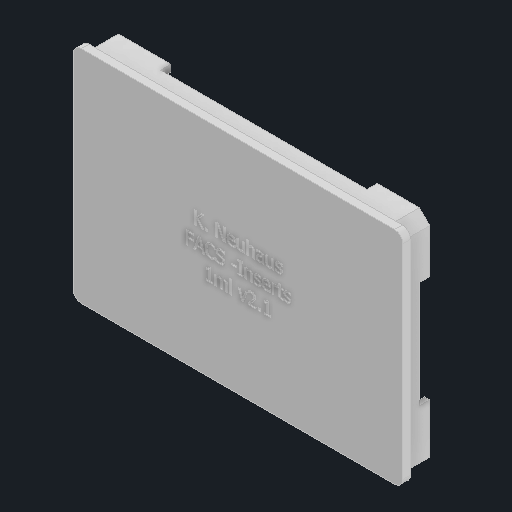
# Autodesk Inventor part: Holder_FACS_1mL_Petridish
Saved by Autodesk Inventor 2026 (Build 300175050, 175E)
## iProperties
Created: 2024-09-30
Part Number: Holder_FACS_1mL_Petridish
Material: Generisch
Document SubType Name: Modeling
Designer: neuhau0004
Density: 1 g/cm^3
Appearance: Vorgabe
Author: neuhau0004
Autodesk Inventor part; units mm, degrees
ref_plane "YZ Plane" through (0, 0, 0) normal (1, 0, 0) x (0, 1, 0)
ref_plane "XZ Plane" through (0, 0, 0) normal (0, 1, 0) x (-1, 0, 0)
ref_plane "XY Plane" through (0, 0, 0) normal (0, 0, 1) x (1, 0, 0)
sketch "Skizze1" plane through (0, 0, 0) normal (0, 0, 1) x (1, 0, 0)
  line L0 (-62.3, -42.74) -> (62.3, -42.74)
  line L1 (62.3, -42.74) -> (62.3, 42.74)
  line L2 (62.3, 42.74) -> (-62.3, 42.74)
  line L3 (-62.3, 42.74) -> (-62.3, -42.74)
  line L4 (-62.3, -42.74) -> (62.3, 42.74) construction
  line L5 (62.3, -42.74) -> (-62.3, 42.74) construction
  line L6 (-60.7, 42.74) -> (60.7, 42.74)
  line L7 (63.88, 39.56) -> (63.88, -39.56)
  line L8 (60.7, -42.74) -> (-60.7, -42.74)
  line L9 (-63.88, -39.56) -> (-63.88, 39.56)
  line L10 (-63.88, 42.74) -> (63.88, -42.74) construction
  line L11 (63.88, 42.74) -> (-63.88, -42.74) construction
  circle A0 centre (-40, 19.74) radius 18.45
  circle A1 centre (0, 19.74) radius 18.45
  circle A2 centre (40, 19.74) radius 18.45
  circle A3 centre (-40, -19.26) radius 18.45
  circle A4 centre (0, -19.26) radius 18.45
  circle A5 centre (40, -19.26) radius 18.45
  arc A6 (63.88, 39.56) -> (60.7, 42.74) centre (60.7, 39.56) ccw
  arc A7 (60.7, -42.74) -> (63.88, -39.56) centre (60.7, -39.56) ccw
  arc A8 (-63.88, -39.56) -> (-60.7, -42.74) centre (-60.7, -39.56) ccw
  arc A9 (-60.7, 42.74) -> (-63.88, 39.56) centre (-60.7, 39.56) ccw
  line L12 (-60.3, 40.85) -> (60.3, 40.85)
  line L13 (60.3, 40.85) -> (60.3, -40.85)
  line L14 (60.3, -40.85) -> (-60.3, -40.85)
  line L15 (-60.3, -40.85) -> (-60.3, 40.85)
  line L16 (-60.3, 40.85) -> (60.3, -40.85) construction
  line L17 (60.3, 40.85) -> (-60.3, -40.85) construction
  ellipse E0 centre (40, 19.74) end of major axis (24, 37.44) minor radius 11.9962
  ellipse E1 centre (0, 19.74) end of major axis (-16, 37.44) minor radius 11.9962
  ellipse E2 centre (-40, 19.74) end of major axis (-56, 37.44) minor radius 11.9962
  ellipse E3 centre (40, -19.26) end of major axis (24, -1.56) minor radius 11.9962
  ellipse E4 centre (0, -19.26) end of major axis (-16, -1.56) minor radius 11.9962
  ellipse E5 centre (-40, -19.26) end of major axis (-56, -1.56) minor radius 11.9962
  line L18 (-40, 40.85) -> (-60.3, 40.85)
  line L19 (-60.3, 40.85) -> (-60.3, 19.74)
  line L20 (-58.45, 19.74) -> (-60.3, 19.74)
  line L21 (-58.45, -19.26) -> (-60.3, -19.26)
  line L22 (-60.3, -40.85) -> (-60.3, -19.26)
  line L23 (-40, -37.71) -> (-40, -40.85)
  line L24 (-60.3, -40.85) -> (-40, -40.85)
  arc A10 (-40, 38.19) -> (-58.45, 19.74) centre (-40, 19.74) ccw
  line L25 (-40, 40.85) -> (-40, 38.19)
  line L26 (40, 38.19) -> (40, 40.85)
  line L27 (58.45, 19.74) -> (60.3, 19.74)
  line L28 (58.45, -19.26) -> (60.3, -19.26)
  line L29 (40, -37.71) -> (40, -40.85)
  line L30 (-60.3, -19.26) -> (-60.3, -21.66)
  line L31 (-60.3, -21.66) -> (-58.2932, -21.66)
  line L32 (60.3, -21.66) -> (58.2932, -21.66)
  point P0 (0, 0)
  point P1 (-60.7, 42.74)
  point P2 (60.7, -42.74)
  point P3 (-22.5977, -25.3889)
  point P4 (-35.6534, -37.1907)
  point P5 (-57.4023, -13.1311)
  point P6 (-44.3466, -1.3293)
  point P7 (17.4023, -25.3889)
  point P8 (4.3466, -37.1907)
  point P9 (-17.4023, -13.1311)
  point P10 (-4.3466, -1.3293)
  point P11 (57.4023, -25.3889)
  point P12 (44.3466, -37.1907)
  point P13 (22.5977, -13.1311)
  point P14 (35.6534, -1.3293)
  point P15 (-22.5977, 13.6111)
  point P16 (-35.6534, 1.8093)
  point P17 (-57.4023, 25.8689)
  point P18 (-44.3466, 37.6707)
  point P19 (17.4023, 13.6111)
  point P20 (4.3466, 1.8093)
  point P21 (-17.4023, 25.8689)
  point P22 (-4.3466, 37.6707)
  point P23 (57.4023, 13.6111)
  point P24 (44.3466, 1.8093)
  point P25 (22.5977, 25.8689)
  point P26 (35.6534, 37.6707)
  point P27 (62.3, 42.3082)
  point P28 (62.3, -42.3082)
  point P29 (-62.3, -42.3082)
  point P30 (-62.3, 42.3082)
  dimension "d0" = 124.6
  dimension "d1" = 85.48
  dimension "d2" = 127.76
  dimension "d3" = 85.48
  dimension "d9" = 36.9
  dimension "d10" = 22.3
  dimension "d13" = 40
  dimension "d16" = 39
  dimension "d19" = 23
  dimension "d20" = 3.18
  dimension "d21" = 3.18
  dimension "d24" = 120.6
  dimension "d25" = 81.7
  dimension "d28" = 40
  dimension "d31" = 39
  dimension "d54" = 2.4
  dimension "d55" = 3.18
  constraints: 66 end point, 20 point on circle, 18 point on line, 13 perpendicular, 11 centre point, 8 tangent, 7 horizontal, 6 midpoint, 6 parallel, 6 vertical, 2 coincident, 2 collinear, 2 equal radius, 27 other
  measures "d0" distance of L2.end L1.end
  measures "d1" distance of L1.end L0.end
  measures "d2" distance of L10.end L11.end
  measures "d3" distance of L11.start L10.end
  measures "d9" diameter of A0
  measures "d10" distance from line of L3 A0.centre
  measures "d13" distance of A0.centre A1.centre
  measures "d16" distance of A0.centre A3.centre
  measures "d19" distance from line of L2 A0.centre
  measures "d20" radius of A6
  measures "d21" radius of A8
  measures "d24" distance of L13.end L14.end
  measures "d25" distance of L12.end L13.end
  measures "d28" distance of point (40, 19.74) point (0, 19.74)
  measures "d31" distance of point (40, 19.74) point (40, -19.26)
  measures "d54" distance of L21.end L30.end
  measures "d55" radius of A9
extrude "Extrusion1" add sketch "Skizze1" along normal blind 3 contours A8 L3 A9 L2 A6 L1 A7 L0 | A8 L9 A9 L3 | L1 A6 L7 A7 | A0 E2 | A0 L25 L12 L26 A2 E0 L27 L13 L28 A5 E3 L29 L14 L23 A3 E5 L21 L15 L20 E2 | A0 E2 L20 L15 L12 L25 | E2 A0 | A0 E2 | A0 E2 | A0 E2 | L12 L13 L27 A2 L26 | A2 E0 | L21 A3 L31 L15 | E0 A2 | A2 E0 | L31 A3 L23 L14 L15 | A3 E5 | L13 L32 A5 L28 | E0 A2 | E0 A2 | E5 A3 | A3 E5 | L13 L14 L29 A5 E3 L32 | A5 E3 | A3 E5 | A3 E5 | E3 A5 | A5 E3 | E3 A5 | E3 A5 | A1 E1 | E1 A1 | A1 E1 | E1 A1 | E1 A1 | A4 E4 | E4 A4 | A4 E4 | E4 A4 | E4 A4
extrude "Extrusion2" add sketch "Skizze1" against normal blind 7 contours A0 L25 L12 L26 A2 E0 L27 L13 L28 A5 E3 L29 L14 L23 A3 E5 L21 L15 L20 E2 | A0 E2 L20 L15 L12 L25 | L12 L13 L27 A2 L26 | L21 A3 L31 L15 | L31 A3 L23 L14 L15 | L13 L32 A5 L28 | L13 L14 L29 A5 E3 L32
fillet "Rundung1" radius 2 3 edges at (60.3, -40.85, -3.5) (-60.3, -40.85, -3.5) (-60.3, 40.85, -3.5)
chamfer "Fase1" distance 1 angle 45 24 edges at (-24, 2.04, -7) (-56, 37.44, -7) (-53.6868, 7.3677, -7) (-26.3132, 32.1123, -7) (-56, -1.56, -7) (-24, -36.96, -7) (-26.3132, -6.8877, -7) (-53.6868, -31.6323, -7) (-16, 37.44, -7) (16, 2.04, -7) (-13.6868, 7.3677, -7) (13.6868, 32.1123, -7) (-16, -1.56, -7) (16, -36.96, -7) (-13.6868, -31.6323, -7) (13.6868, -6.8877, -7) (24, 37.44, -7) (56, 2.04, -7) (26.3132, 7.3677, -7) (53.6868, 32.1123, -7) (24, -1.56, -7) (56, -36.96, -7) (53.6868, -6.8877, -7) (26.3132, -31.6323, -7)
chamfer "Fase2" distance 4 angle 45 1 edges at (60.3, 40.85, -3.5)
sketch "Skizze3" plane through (0, 0, 3) normal (0, 0, 1) x (1, 0, 0)
  line L0 (-25.4173, 12.5) -> (25.4173, 12.5) construction
  line L1 (25.4173, 12.5) -> (25.4173, -12.5) construction
  line L2 (25.4173, -12.5) -> (-25.4173, -12.5) construction
  line L3 (-25.4173, -12.5) -> (-25.4173, 12.5) construction
  line L4 (-13.1767, 5.6209) -> (-14.0397, 5.6209)
  line L5 (-14.0397, 5.6209) -> (-15.8671, 7.9467)
  line L6 (-15.8671, 7.9467) -> (-16.1588, 7.6185)
  line L7 (-16.1588, 7.6185) -> (-16.1588, 5.6209)
  line L8 (-16.1588, 5.6209) -> (-16.8233, 5.6209)
  line L9 (-16.8233, 5.6209) -> (-16.8233, 10.6209)
  line L10 (-16.8233, 10.6209) -> (-16.1588, 10.6209)
  line L11 (-16.1588, 10.6209) -> (-16.1588, 8.3235)
  line L12 (-16.1588, 8.3235) -> (-14.1086, 10.6209)
  line L13 (-14.1086, 10.6209) -> (-13.2982, 10.6209)
  line L14 (-13.2982, 10.6209) -> (-15.3687, 8.3884)
  line L15 (-15.3687, 8.3884) -> (-13.1767, 5.6209)
  line L16 (-11.8476, 5.6209) -> (-12.6499, 5.6209)
  line L17 (-12.6499, 5.6209) -> (-12.6499, 6.5772)
  line L18 (-12.6499, 6.5772) -> (-11.8476, 6.5772)
  line L19 (-11.8476, 6.5772) -> (-11.8476, 5.6209)
  line L20 (-4.9716, 5.6209) -> (-5.7172, 5.6209)
  line L21 (-5.7172, 5.6209) -> (-7.9295, 9.9321)
  line L22 (-7.9295, 9.9321) -> (-7.9295, 5.6209)
  line L23 (-7.9295, 5.6209) -> (-8.5494, 5.6209)
  line L24 (-8.5494, 5.6209) -> (-8.5494, 10.6209)
  line L25 (-8.5494, 10.6209) -> (-7.6053, 10.6209)
  line L26 (-7.6053, 10.6209) -> (-5.5916, 6.6623)
  line L27 (-5.5916, 6.6623) -> (-5.5916, 10.6209)
  line L28 (-5.5916, 10.6209) -> (-4.9716, 10.6209)
  line L29 (-4.9716, 10.6209) -> (-4.9716, 5.6209)
  spline S0 degree 2 poles (-2.3784, 5.5359) (-3.278, 5.5359) (-4.2666, 6.5448) (-4.2666, 7.4767) knots 0 0 0 1 2 2 2
  spline S1 degree 2 poles (-4.2666, 7.4767) (-4.2666, 8.3924) (-3.3063, 9.4783) (-2.5324, 9.4783) knots 0 0 0 1 2 2 2
  spline S2 degree 2 poles (-2.5324, 9.4783) (-2.184, 9.4783) (-1.6451, 9.2757) (-1.4465, 9.061) knots 0 0 0 1 2 2 2
  spline S3 degree 2 poles (-1.4465, 9.061) (-1.2439, 8.8462) (-1.0292, 8.2263) (-1.0292, 7.7765) knots 0 0 0 1 2 2 2
  line L30 (-1.0292, 7.7765) -> (-1.0292, 7.4321)
  line L31 (-1.0292, 7.4321) -> (-3.6264, 7.4321)
  spline S4 degree 2 poles (-3.6264, 7.4321) (-3.6264, 6.7798) (-2.97, 6.0869) (-2.3865, 6.0869) knots 0 0 0 1 2 2 2
  spline S5 degree 2 poles (-2.3865, 6.0869) (-2.1799, 6.0869) (-1.7788, 6.1801) (-1.6167, 6.253) knots 0 0 0 1 2 2 2
  spline S6 degree 2 poles (-1.6167, 6.253) (-1.4465, 6.3341) (-1.2115, 6.4759) (-1.1345, 6.5407) knots 0 0 0 1 2 2 2
  line L32 (-1.1345, 6.5407) -> (-1.0981, 6.5407)
  line L33 (-1.0981, 6.5407) -> (-1.0981, 5.8519)
  spline S7 degree 2 poles (-1.0981, 5.8519) (-1.2075, 5.8073) (-1.5397, 5.6777) (-1.6694, 5.6412) knots 0 0 0 1 2 2 2
  spline S8 degree 2 poles (-1.6694, 5.6412) (-1.8517, 5.5885) (-2.1515, 5.5359) (-2.3784, 5.5359) knots 0 0 0 1 2 2 2
  spline S9 degree 2 poles (-1.6451, 7.9143) (-1.6532, 8.1696) (-1.7585, 8.5423) (-1.8598, 8.6679) knots 0 0 0 1 2 2 2
  spline S10 degree 2 poles (-1.8598, 8.6679) (-1.9692, 8.8098) (-2.3136, 8.9597) (-2.5689, 8.9597) knots 0 0 0 1 2 2 2
  spline S11 degree 2 poles (-2.5689, 8.9597) (-2.8201, 8.9597) (-3.1726, 8.8098) (-3.3185, 8.6639) knots 0 0 0 1 2 2 2
  spline S12 degree 2 poles (-3.3185, 8.6639) (-3.4603, 8.514) (-3.6062, 8.1534) (-3.6264, 7.9143) knots 0 0 0 1 2 2 2
  line L34 (-3.6264, 7.9143) -> (-1.6451, 7.9143)
  line L35 (2.5284, 5.6209) -> (1.8963, 5.6209)
  line L36 (1.8963, 5.6209) -> (1.8963, 6.0342)
  spline S13 degree 2 poles (1.8963, 6.0342) (1.6045, 5.779) (1.0818, 5.5156) (0.7577, 5.5156) knots 0 0 0 1 2 2 2
  spline S14 degree 2 poles (0.7577, 5.5156) (0.5146, 5.5156) (0.081, 5.6777) (-0.077, 5.8519) knots 0 0 0 1 2 2 2
  spline S15 degree 2 poles (-0.077, 5.8519) (-0.2391, 6.0261) (-0.4173, 6.5569) (-0.4173, 6.9378) knots 0 0 0 1 2 2 2
  line L37 (-0.4173, 6.9378) -> (-0.4173, 9.373)
  line L38 (-0.4173, 9.373) -> (0.2147, 9.373)
  line L39 (0.2147, 9.373) -> (0.2147, 7.2336)
  spline S16 degree 2 poles (0.2147, 7.2336) (0.2147, 6.9337) (0.2593, 6.5407) (0.3363, 6.3948) knots 0 0 0 1 2 2 2
  spline S17 degree 2 poles (0.3363, 6.3948) (0.4133, 6.249) (0.6767, 6.1153) (0.9238, 6.1153) knots 0 0 0 1 2 2 2
  spline S18 degree 2 poles (0.9238, 6.1153) (1.1548, 6.1153) (1.6775, 6.3786) (1.8963, 6.5691) knots 0 0 0 1 2 2 2
  line L40 (1.8963, 6.5691) -> (1.8963, 9.373)
  line L41 (1.8963, 9.373) -> (2.5284, 9.373)
  line L42 (2.5284, 9.373) -> (2.5284, 5.6209)
  line L43 (6.3898, 5.6209) -> (5.7577, 5.6209)
  line L44 (5.7577, 5.6209) -> (5.7577, 7.7603)
  spline S19 degree 2 poles (5.7577, 7.7603) (5.7577, 8.0196) (5.7091, 8.4654) (5.6361, 8.5991) knots 0 0 0 1 2 2 2
  spline S20 degree 2 poles (5.6361, 8.5991) (5.5592, 8.7409) (5.2836, 8.8786) (5.0486, 8.8786) knots 0 0 0 1 2 2 2
  spline S21 degree 2 poles (5.0486, 8.8786) (4.8136, 8.8786) (4.3152, 8.6274) (4.0762, 8.4248) knots 0 0 0 1 2 2 2
  line L45 (4.0762, 8.4248) -> (4.0762, 5.6209)
  line L46 (4.0762, 5.6209) -> (3.4441, 5.6209)
  line L47 (3.4441, 5.6209) -> (3.4441, 10.8438)
  line L48 (3.4441, 10.8438) -> (4.0762, 10.8438)
  line L49 (4.0762, 10.8438) -> (4.0762, 8.9556)
  spline S22 degree 2 poles (4.0762, 8.9556) (4.3598, 9.2109) (4.9068, 9.4783) (5.2147, 9.4783) knots 0 0 0 1 2 2 2
  spline S23 degree 2 poles (5.2147, 9.4783) (5.7658, 9.4783) (6.3898, 8.749) (6.3898, 8.0561) knots 0 0 0 1 2 2 2
  line L50 (6.3898, 8.0561) -> (6.3898, 5.6209)
  spline S24 degree 2 poles (9.3679, 6.018) (9.2909, 5.9613) (9.0316, 5.7587) (8.91, 5.6979) knots 0 0 0 1 2 2 2
  spline S25 degree 2 poles (8.91, 5.6979) (8.7439, 5.6088) (8.4319, 5.5156) (8.1483, 5.5156) knots 0 0 0 1 2 2 2
  spline S26 degree 2 poles (8.1483, 5.5156) (7.9173, 5.5156) (7.5, 5.6898) (7.342, 5.8478) knots 0 0 0 1 2 2 2
  spline S27 degree 2 poles (7.342, 5.8478) (7.1921, 6.0018) (7.0097, 6.4556) (7.0097, 6.7068) knots 0 0 0 1 2 2 2
  spline S28 degree 2 poles (7.0097, 6.7068) (7.0097, 7.0958) (7.3379, 7.6469) (7.6945, 7.8049) knots 0 0 0 1 2 2 2
  spline S29 degree 2 poles (7.6945, 7.8049) (8.0105, 7.9508) (8.8695, 8.0602) (9.3679, 8.0885) knots 0 0 0 1 2 2 2
  line L51 (9.3679, 8.0885) -> (9.3679, 8.2101)
  spline S30 degree 2 poles (9.3679, 8.2101) (9.3679, 8.4289) (9.2342, 8.7004) (9.1126, 8.7773) knots 0 0 0 1 2 2 2
  spline S31 degree 2 poles (9.1126, 8.7773) (8.9911, 8.8543) (8.6426, 8.903) (8.4562, 8.903) knots 0 0 0 1 2 2 2
  spline S32 degree 2 poles (8.4562, 8.903) (8.2374, 8.903) (7.6459, 8.7733) (7.3501, 8.6477) knots 0 0 0 1 2 2 2
  line L52 (7.3501, 8.6477) -> (7.3136, 8.6477)
  line L53 (7.3136, 8.6477) -> (7.3136, 9.2919)
  spline S33 degree 2 poles (7.3136, 9.2919) (7.4878, 9.3406) (8.1402, 9.4621) (8.4603, 9.4621) knots 0 0 0 1 2 2 2
  spline S34 degree 2 poles (8.4603, 9.4621) (8.8493, 9.4621) (9.3801, 9.3406) (9.5908, 9.1825) knots 0 0 0 1 2 2 2
  spline S35 degree 2 poles (9.5908, 9.1825) (9.7974, 9.0286) (10, 8.5383) (10, 8.1858) knots 0 0 0 1 2 2 2
  line L54 (10, 8.1858) -> (10, 5.6209)
  line L55 (10, 5.6209) -> (9.3679, 5.6209)
  line L56 (9.3679, 5.6209) -> (9.3679, 6.018)
  line L57 (9.3679, 6.5448) -> (9.3679, 7.5861)
  spline S36 degree 2 poles (9.3679, 7.5861) (9.141, 7.5658) (8.4562, 7.497) (8.2415, 7.4321) knots 0 0 0 1 2 2 2
  spline S37 degree 2 poles (8.2415, 7.4321) (7.9903, 7.3551) (7.6621, 7.035) (7.6621, 6.7514) knots 0 0 0 1 2 2 2
  spline S38 degree 2 poles (7.6621, 6.7514) (7.6621, 6.4273) (8.0267, 6.0991) (8.3752, 6.0991) knots 0 0 0 1 2 2 2
  spline S39 degree 2 poles (8.3752, 6.0991) (8.671, 6.0991) (9.1572, 6.3543) (9.3679, 6.5448) knots 0 0 0 1 2 2 2
  line L58 (13.8047, 5.6209) -> (13.1726, 5.6209)
  line L59 (13.1726, 5.6209) -> (13.1726, 6.0342)
  spline S40 degree 2 poles (13.1726, 6.0342) (12.8809, 5.779) (12.3582, 5.5156) (12.034, 5.5156) knots 0 0 0 1 2 2 2
  spline S41 degree 2 poles (12.034, 5.5156) (11.7909, 5.5156) (11.3574, 5.6777) (11.1994, 5.8519) knots 0 0 0 1 2 2 2
  spline S42 degree 2 poles (11.1994, 5.8519) (11.0373, 6.0261) (10.859, 6.5569) (10.859, 6.9378) knots 0 0 0 1 2 2 2
  line L60 (10.859, 6.9378) -> (10.859, 9.373)
  line L61 (10.859, 9.373) -> (11.4911, 9.373)
  line L62 (11.4911, 9.373) -> (11.4911, 7.2336)
  spline S43 degree 2 poles (11.4911, 7.2336) (11.4911, 6.9337) (11.5357, 6.5407) (11.6126, 6.3948) knots 0 0 0 1 2 2 2
  spline S44 degree 2 poles (11.6126, 6.3948) (11.6896, 6.249) (11.953, 6.1153) (12.2002, 6.1153) knots 0 0 0 1 2 2 2
  spline S45 degree 2 poles (12.2002, 6.1153) (12.4311, 6.1153) (12.9538, 6.3786) (13.1726, 6.5691) knots 0 0 0 1 2 2 2
  line L63 (13.1726, 6.5691) -> (13.1726, 9.373)
  line L64 (13.1726, 9.373) -> (13.8047, 9.373)
  line L65 (13.8047, 9.373) -> (13.8047, 5.6209)
  spline S46 degree 2 poles (15.7334, 5.5318) (15.3566, 5.5318) (14.7042, 5.7344) (14.4895, 5.8478) knots 0 0 0 1 2 2 2
  line L66 (14.4895, 5.8478) -> (14.4895, 6.5569)
  line L67 (14.4895, 6.5569) -> (14.5219, 6.5569)
  spline S47 degree 2 poles (14.5219, 6.5569) (14.6029, 6.4921) (14.8217, 6.3381) (15.0041, 6.253) knots 0 0 0 1 2 2 2
  spline S48 degree 2 poles (15.0041, 6.253) (15.1621, 6.176) (15.5511, 6.0626) (15.7577, 6.0626) knots 0 0 0 1 2 2 2
  spline S49 degree 2 poles (15.7577, 6.0626) (15.9076, 6.0626) (16.252, 6.1315) (16.3331, 6.1882) knots 0 0 0 1 2 2 2
  spline S50 degree 2 poles (16.3331, 6.1882) (16.4506, 6.2652) (16.5559, 6.4394) (16.5559, 6.6177) knots 0 0 0 1 2 2 2
  spline S51 degree 2 poles (16.5559, 6.6177) (16.5559, 6.8406) (16.3128, 7.0715) (16.0008, 7.1485) knots 0 0 0 1 2 2 2
  spline S52 degree 2 poles (16.0008, 7.1485) (15.8793, 7.1769) (15.4903, 7.2579) (15.3241, 7.3025) knots 0 0 0 1 2 2 2
  spline S53 degree 2 poles (15.3241, 7.3025) (14.8947, 7.4281) (14.5057, 7.9467) (14.5057, 8.3154) knots 0 0 0 1 2 2 2
  spline S54 degree 2 poles (14.5057, 8.3154) (14.5057, 8.826) (15.2715, 9.4621) (15.9036, 9.4621) knots 0 0 0 1 2 2 2
  spline S55 degree 2 poles (15.9036, 9.4621) (16.2156, 9.4621) (16.8477, 9.3081) (17.0624, 9.1906) knots 0 0 0 1 2 2 2
  line L68 (17.0624, 9.1906) -> (17.0624, 8.514)
  line L69 (17.0624, 8.514) -> (17.03, 8.514)
  spline S56 degree 2 poles (17.03, 8.514) (16.7869, 8.7085) (16.1953, 8.9313) (15.8914, 8.9313) knots 0 0 0 1 2 2 2
  spline S57 degree 2 poles (15.8914, 8.9313) (15.5794, 8.9313) (15.1499, 8.6679) (15.1499, 8.4046) knots 0 0 0 1 2 2 2
  spline S58 degree 2 poles (15.1499, 8.4046) (15.1499, 8.1655) (15.4052, 7.9346) (15.6888, 7.8616) knots 0 0 0 1 2 2 2
  spline S59 degree 2 poles (15.6888, 7.8616) (15.8266, 7.8252) (16.175, 7.7522) (16.3655, 7.7077) knots 0 0 0 1 2 2 2
  spline S60 degree 2 poles (16.3655, 7.7077) (16.7788, 7.6023) (17.2002, 7.1201) (17.2002, 6.7028) knots 0 0 0 1 2 2 2
  spline S61 degree 2 poles (17.2002, 6.7028) (17.2002, 6.4597) (17.0097, 6.0302) (16.8233, 5.8722) knots 0 0 0 1 2 2 2
  spline S62 degree 2 poles (16.8233, 5.8722) (16.6248, 5.706) (16.1183, 5.5318) (15.7334, 5.5318) knots 0 0 0 1 2 2 2
  line L70 (-17.1252, 1.797) -> (-19.451, 1.797)
  line L71 (-19.451, 1.797) -> (-19.451, 0.387)
  line L72 (-19.451, 0.387) -> (-17.2224, 0.387)
  line L73 (-17.2224, 0.387) -> (-17.2224, -0.2046)
  line L74 (-17.2224, -0.2046) -> (-19.451, -0.2046)
  line L75 (-19.451, -0.2046) -> (-19.451, -2.6114)
  line L76 (-19.451, -2.6114) -> (-20.1155, -2.6114)
  line L77 (-20.1155, -2.6114) -> (-20.1155, 2.3886)
  line L78 (-20.1155, 2.3886) -> (-17.1252, 2.3886)
  line L79 (-17.1252, 2.3886) -> (-17.1252, 1.797)
  line L80 (-17.0685, -2.6114) -> (-15.3829, 2.3886)
  line L81 (-15.3829, 2.3886) -> (-14.5644, 2.3886)
  line L82 (-14.5644, 2.3886) -> (-12.8788, -2.6114)
  line L83 (-12.8788, -2.6114) -> (-13.5798, -2.6114)
  line L84 (-13.5798, -2.6114) -> (-14.0336, -1.2135)
  line L85 (-14.0336, -1.2135) -> (-15.9421, -1.2135)
  line L86 (-15.9421, -1.2135) -> (-16.3959, -2.6114)
  line L87 (-16.3959, -2.6114) -> (-17.0685, -2.6114)
  line L88 (-14.216, -0.6463) -> (-14.9899, 1.7079)
  line L89 (-14.9899, 1.7079) -> (-15.7597, -0.6463)
  line L90 (-15.7597, -0.6463) -> (-14.216, -0.6463)
  spline S63 degree 2 poles (-10.4518, -2.7006) (-10.938, -2.7006) (-11.7605, -2.3724) (-12.0604, -2.0442) knots 0 0 0 1 2 2 2
  spline S64 degree 2 poles (-12.0604, -2.0442) (-12.3602, -1.72) (-12.6884, -0.7476) (-12.6884, -0.1155) knots 0 0 0 1 2 2 2
  spline S65 degree 2 poles (-12.6884, -0.1155) (-12.6884, 0.5126) (-12.3683, 1.4445) (-12.0644, 1.7889) knots 0 0 0 1 2 2 2
  spline S66 degree 2 poles (-12.0644, 1.7889) (-11.7646, 2.1252) (-10.9461, 2.4777) (-10.4396, 2.4777) knots 0 0 0 1 2 2 2
  spline S67 degree 2 poles (-10.4396, 2.4777) (-10.1884, 2.4777) (-9.7468, 2.4048) (-9.5604, 2.3481) knots 0 0 0 1 2 2 2
  spline S68 degree 2 poles (-9.5604, 2.3481) (-9.3983, 2.2954) (-9.062, 2.1455) (-8.8959, 2.0563) knots 0 0 0 1 2 2 2
  line L91 (-8.8959, 2.0563) -> (-8.8959, 1.2541)
  line L92 (-8.8959, 1.2541) -> (-8.9485, 1.2541)
  spline S69 degree 2 poles (-8.9485, 1.2541) (-9.0377, 1.3351) (-9.3132, 1.562) (-9.5117, 1.6714) knots 0 0 0 1 2 2 2
  spline S70 degree 2 poles (-9.5117, 1.6714) (-9.7022, 1.7767) (-10.1519, 1.9105) (-10.4437, 1.9105) knots 0 0 0 1 2 2 2
  spline S71 degree 2 poles (-10.4437, 1.9105) (-10.7638, 1.9105) (-11.3351, 1.6471) (-11.5498, 1.3959) knots 0 0 0 1 2 2 2
  spline S72 degree 2 poles (-11.5498, 1.3959) (-11.7605, 1.1406) (-11.9955, 0.3667) (-11.9955, -0.1155) knots 0 0 0 1 2 2 2
  spline S73 degree 2 poles (-11.9955, -0.1155) (-11.9955, -0.6301) (-11.7484, -1.3716) (-11.5336, -1.6268) knots 0 0 0 1 2 2 2
  spline S74 degree 2 poles (-11.5336, -1.6268) (-11.3229, -1.874) (-10.7597, -2.1252) (-10.4437, -2.1252) knots 0 0 0 1 2 2 2
  spline S75 degree 2 poles (-10.4437, -2.1252) (-10.156, -2.1252) (-9.6657, -1.9834) (-9.4753, -1.878) knots 0 0 0 1 2 2 2
  spline S76 degree 2 poles (-9.4753, -1.878) (-9.2929, -1.7727) (-9.0215, -1.5539) (-8.9445, -1.4769) knots 0 0 0 1 2 2 2
  line L93 (-8.9445, -1.4769) -> (-8.8959, -1.4769)
  line L94 (-8.8959, -1.4769) -> (-8.8959, -2.2711)
  spline S77 degree 2 poles (-8.8959, -2.2711) (-9.062, -2.3481) (-9.3537, -2.4899) (-9.5604, -2.5547) knots 0 0 0 1 2 2 2
  spline S78 degree 2 poles (-9.5604, -2.5547) (-9.7792, -2.6276) (-10.1519, -2.7006) (-10.4518, -2.7006) knots 0 0 0 1 2 2 2
  spline S79 degree 2 poles (-6.8821, -2.7006) (-7.425, -2.7006) (-8.1868, -2.4737) (-8.5231, -2.3116) knots 0 0 0 1 2 2 2
  line L95 (-8.5231, -2.3116) -> (-8.5231, -1.4769)
  line L96 (-8.5231, -1.4769) -> (-8.4745, -1.4769)
  spline S80 degree 2 poles (-8.4745, -1.4769) (-8.1463, -1.7848) (-7.3156, -2.1252) (-6.9307, -2.1252) knots 0 0 0 1 2 2 2
  spline S81 degree 2 poles (-6.9307, -2.1252) (-6.3797, -2.1252) (-5.8164, -1.6673) (-5.8164, -1.2905) knots 0 0 0 1 2 2 2
  spline S82 degree 2 poles (-5.8164, -1.2905) (-5.8164, -0.9907) (-6.1122, -0.6179) (-6.4323, -0.5247) knots 0 0 0 1 2 2 2
  spline S83 degree 2 poles (-6.4323, -0.5247) (-6.6633, -0.4599) (-7.0482, -0.3707) (-7.3359, -0.2978) knots 0 0 0 1 2 2 2
  spline S84 degree 2 poles (-7.3359, -0.2978) (-7.5952, -0.2289) (-8.0045, -0.0223) (-8.1625, 0.1438) knots 0 0 0 1 2 2 2
  spline S85 degree 2 poles (-8.1625, 0.1438) (-8.3164, 0.31) (-8.4866, 0.7557) (-8.4866, 1.0474) knots 0 0 0 1 2 2 2
  spline S86 degree 2 poles (-8.4866, 1.0474) (-8.4866, 1.6552) (-7.5385, 2.4777) (-6.8051, 2.4777) knots 0 0 0 1 2 2 2
  spline S87 degree 2 poles (-6.8051, 2.4777) (-6.3837, 2.4777) (-5.6382, 2.3116) (-5.3181, 2.1536) knots 0 0 0 1 2 2 2
  line L97 (-5.3181, 2.1536) -> (-5.3181, 1.3594)
  line L98 (-5.3181, 1.3594) -> (-5.3667, 1.3594)
  spline S88 degree 2 poles (-5.3667, 1.3594) (-5.6058, 1.5782) (-6.3513, 1.9024) (-6.7605, 1.9024) knots 0 0 0 1 2 2 2
  spline S89 degree 2 poles (-6.7605, 1.9024) (-7.2224, 1.9024) (-7.7938, 1.4688) (-7.7938, 1.1163) knots 0 0 0 1 2 2 2
  spline S90 degree 2 poles (-7.7938, 1.1163) (-7.7938, 0.8002) (-7.4575, 0.4234) (-7.1414, 0.3383) knots 0 0 0 1 2 2 2
  spline S91 degree 2 poles (-7.1414, 0.3383) (-6.9307, 0.2816) (-6.3189, 0.1357) (-6.1163, 0.075) knots 0 0 0 1 2 2 2
  spline S92 degree 2 poles (-6.1163, 0.075) (-5.6017, -0.0831) (-5.1236, -0.7192) (-5.1236, -1.1852) knots 0 0 0 1 2 2 2
  spline S93 degree 2 poles (-5.1236, -1.1852) (-5.1236, -1.481) (-5.3626, -2.0482) (-5.5774, -2.2468) knots 0 0 0 1 2 2 2
  spline S94 degree 2 poles (-5.5774, -2.2468) (-5.8164, -2.4656) (-6.4242, -2.7006) (-6.8821, -2.7006) knots 0 0 0 1 2 2 2
  line L99 (-0.6098, -0.7273) -> (-2.502, -0.7273)
  line L100 (-2.502, -0.7273) -> (-2.502, -0.1195)
  line L101 (-2.502, -0.1195) -> (-0.6098, -0.1195)
  line L102 (-0.6098, -0.1195) -> (-0.6098, -0.7273)
  line L103 (1.9388, -2.6114) -> (0.002, -2.6114)
  line L104 (0.002, -2.6114) -> (0.002, -2.1009)
  line L105 (0.002, -2.1009) -> (0.6382, -2.1009)
  line L106 (0.6382, -2.1009) -> (0.6382, 1.878)
  line L107 (0.6382, 1.878) -> (0.002, 1.878)
  line L108 (0.002, 1.878) -> (0.002, 2.3886)
  line L109 (0.002, 2.3886) -> (1.9388, 2.3886)
  line L110 (1.9388, 2.3886) -> (1.9388, 1.878)
  line L111 (1.9388, 1.878) -> (1.3027, 1.878)
  line L112 (1.3027, 1.878) -> (1.3027, -2.1009)
  line L113 (1.3027, -2.1009) -> (1.9388, -2.1009)
  line L114 (1.9388, -2.1009) -> (1.9388, -2.6114)
  line L115 (5.6584, -2.6114) -> (5.0263, -2.6114)
  line L116 (5.0263, -2.6114) -> (5.0263, -0.472)
  spline S95 degree 2 poles (5.0263, -0.472) (5.0263, -0.2127) (4.9777, 0.233) (4.9048, 0.3667) knots 0 0 0 1 2 2 2
  spline S96 degree 2 poles (4.9048, 0.3667) (4.8278, 0.5085) (4.5523, 0.6463) (4.3173, 0.6463) knots 0 0 0 1 2 2 2
  spline S97 degree 2 poles (4.3173, 0.6463) (4.0823, 0.6463) (3.5839, 0.3951) (3.3448, 0.1925) knots 0 0 0 1 2 2 2
  line L117 (3.3448, 0.1925) -> (3.3448, -2.6114)
  line L118 (3.3448, -2.6114) -> (2.7127, -2.6114)
  line L119 (2.7127, -2.6114) -> (2.7127, 1.1406)
  line L120 (2.7127, 1.1406) -> (3.3448, 1.1406)
  line L121 (3.3448, 1.1406) -> (3.3448, 0.7233)
  spline S98 degree 2 poles (3.3448, 0.7233) (3.6284, 0.9785) (4.1754, 1.2459) (4.4834, 1.2459) knots 0 0 0 1 2 2 2
  spline S99 degree 2 poles (4.4834, 1.2459) (5.0344, 1.2459) (5.6584, 0.5166) (5.6584, -0.1763) knots 0 0 0 1 2 2 2
  line L122 (5.6584, -0.1763) -> (5.6584, -2.6114)
  spline S100 degree 2 poles (7.5588, -2.7006) (7.1819, -2.7006) (6.5296, -2.498) (6.3148, -2.3845) knots 0 0 0 1 2 2 2
  line L123 (6.3148, -2.3845) -> (6.3148, -1.6754)
  line L124 (6.3148, -1.6754) -> (6.3472, -1.6754)
  spline S101 degree 2 poles (6.3472, -1.6754) (6.4283, -1.7403) (6.6471, -1.8942) (6.8294, -1.9793) knots 0 0 0 1 2 2 2
  spline S102 degree 2 poles (6.8294, -1.9793) (6.9874, -2.0563) (7.3764, -2.1698) (7.5831, -2.1698) knots 0 0 0 1 2 2 2
  spline S103 degree 2 poles (7.5831, -2.1698) (7.733, -2.1698) (8.0774, -2.1009) (8.1584, -2.0442) knots 0 0 0 1 2 2 2
  spline S104 degree 2 poles (8.1584, -2.0442) (8.2759, -1.9672) (8.3813, -1.7929) (8.3813, -1.6147) knots 0 0 0 1 2 2 2
  spline S105 degree 2 poles (8.3813, -1.6147) (8.3813, -1.3918) (8.1382, -1.1609) (7.8262, -1.0839) knots 0 0 0 1 2 2 2
  spline S106 degree 2 poles (7.8262, -1.0839) (7.7046, -1.0555) (7.3156, -0.9745) (7.1495, -0.9299) knots 0 0 0 1 2 2 2
  spline S107 degree 2 poles (7.1495, -0.9299) (6.72, -0.8043) (6.331, -0.2857) (6.331, 0.0831) knots 0 0 0 1 2 2 2
  spline S108 degree 2 poles (6.331, 0.0831) (6.331, 0.5936) (7.0968, 1.2297) (7.7289, 1.2297) knots 0 0 0 1 2 2 2
  spline S109 degree 2 poles (7.7289, 1.2297) (8.0409, 1.2297) (8.673, 1.0758) (8.8878, 0.9583) knots 0 0 0 1 2 2 2
  line L125 (8.8878, 0.9583) -> (8.8878, 0.2816)
  line L126 (8.8878, 0.2816) -> (8.8553, 0.2816)
  spline S110 degree 2 poles (8.8553, 0.2816) (8.6122, 0.4761) (8.0207, 0.6989) (7.7168, 0.6989) knots 0 0 0 1 2 2 2
  spline S111 degree 2 poles (7.7168, 0.6989) (7.4048, 0.6989) (6.9753, 0.4356) (6.9753, 0.1722) knots 0 0 0 1 2 2 2
  spline S112 degree 2 poles (6.9753, 0.1722) (6.9753, -0.0669) (7.2306, -0.2978) (7.5142, -0.3707) knots 0 0 0 1 2 2 2
  spline S113 degree 2 poles (7.5142, -0.3707) (7.6519, -0.4072) (8.0004, -0.4801) (8.1908, -0.5247) knots 0 0 0 1 2 2 2
  spline S114 degree 2 poles (8.1908, -0.5247) (8.6041, -0.6301) (9.0255, -1.1122) (9.0255, -1.5296) knots 0 0 0 1 2 2 2
  spline S115 degree 2 poles (9.0255, -1.5296) (9.0255, -1.7727) (8.8351, -2.2022) (8.6487, -2.3602) knots 0 0 0 1 2 2 2
  spline S116 degree 2 poles (8.6487, -2.3602) (8.4502, -2.5263) (7.9437, -2.7006) (7.5588, -2.7006) knots 0 0 0 1 2 2 2
  spline S117 degree 2 poles (11.2419, -2.6965) (10.3424, -2.6965) (9.3537, -1.6876) (9.3537, -0.7557) knots 0 0 0 1 2 2 2
  spline S118 degree 2 poles (9.3537, -0.7557) (9.3537, 0.16) (10.314, 1.2459) (11.0879, 1.2459) knots 0 0 0 1 2 2 2
  spline S119 degree 2 poles (11.0879, 1.2459) (11.4364, 1.2459) (11.9753, 1.0434) (12.1738, 0.8286) knots 0 0 0 1 2 2 2
  spline S120 degree 2 poles (12.1738, 0.8286) (12.3764, 0.6139) (12.5912, -0.0061) (12.5912, -0.4558) knots 0 0 0 1 2 2 2
  line L127 (12.5912, -0.4558) -> (12.5912, -0.8002)
  line L128 (12.5912, -0.8002) -> (9.9939, -0.8002)
  spline S121 degree 2 poles (9.9939, -0.8002) (9.9939, -1.4526) (10.6503, -2.1455) (11.2338, -2.1455) knots 0 0 0 1 2 2 2
  spline S122 degree 2 poles (11.2338, -2.1455) (11.4404, -2.1455) (11.8416, -2.0523) (12.0036, -1.9793) knots 0 0 0 1 2 2 2
  spline S123 degree 2 poles (12.0036, -1.9793) (12.1738, -1.8983) (12.4088, -1.7565) (12.4858, -1.6917) knots 0 0 0 1 2 2 2
  line L129 (12.4858, -1.6917) -> (12.5223, -1.6917)
  line L130 (12.5223, -1.6917) -> (12.5223, -2.3805)
  spline S124 degree 2 poles (12.5223, -2.3805) (12.4129, -2.425) (12.0806, -2.5547) (11.951, -2.5912) knots 0 0 0 1 2 2 2
  spline S125 degree 2 poles (11.951, -2.5912) (11.7686, -2.6438) (11.4688, -2.6965) (11.2419, -2.6965) knots 0 0 0 1 2 2 2
  spline S126 degree 2 poles (11.9753, -0.3181) (11.9672, -0.0628) (11.8618, 0.31) (11.7605, 0.4356) knots 0 0 0 1 2 2 2
  spline S127 degree 2 poles (11.7605, 0.4356) (11.6511, 0.5774) (11.3067, 0.7273) (11.0515, 0.7273) knots 0 0 0 1 2 2 2
  spline S128 degree 2 poles (11.0515, 0.7273) (10.8002, 0.7273) (10.4477, 0.5774) (10.3019, 0.4315) knots 0 0 0 1 2 2 2
  spline S129 degree 2 poles (10.3019, 0.4315) (10.16, 0.2816) (10.0142, -0.079) (9.9939, -0.3181) knots 0 0 0 1 2 2 2
  line L131 (9.9939, -0.3181) -> (11.9753, -0.3181)
  line L132 (15.2208, 0.4639) -> (15.1884, 0.4639)
  spline S130 degree 2 poles (15.1884, 0.4639) (15.1155, 0.4842) (14.9575, 0.4923) (14.8481, 0.4923) knots 0 0 0 1 2 2 2
  spline S131 degree 2 poles (14.8481, 0.4923) (14.5928, 0.4923) (14.0904, 0.2694) (13.8635, 0.0506) knots 0 0 0 1 2 2 2
  line L133 (13.8635, 0.0506) -> (13.8635, -2.6114)
  line L134 (13.8635, -2.6114) -> (13.2314, -2.6114)
  line L135 (13.2314, -2.6114) -> (13.2314, 1.1406)
  line L136 (13.2314, 1.1406) -> (13.8635, 1.1406)
  line L137 (13.8635, 1.1406) -> (13.8635, 0.5814)
  spline S132 degree 2 poles (13.8635, 0.5814) (14.2079, 0.8894) (14.7224, 1.1406) (14.9656, 1.1406) knots 0 0 0 1 2 2 2
  spline S133 degree 2 poles (14.9656, 1.1406) (15.0628, 1.1406) (15.16, 1.1325) (15.2208, 1.1203) knots 0 0 0 1 2 2 2
  line L138 (15.2208, 1.1203) -> (15.2208, 0.4639)
  spline S134 degree 2 poles (16.8456, -2.6844) (16.331, -2.6844) (15.7516, -2.0968) (15.7516, -1.4607) knots 0 0 0 1 2 2 2
  line L139 (15.7516, -1.4607) -> (15.7516, 0.6179)
  line L140 (15.7516, 0.6179) -> (15.3262, 0.6179)
  line L141 (15.3262, 0.6179) -> (15.3262, 1.1406)
  line L142 (15.3262, 1.1406) -> (15.7516, 1.1406)
  line L143 (15.7516, 1.1406) -> (15.7516, 2.2184)
  line L144 (15.7516, 2.2184) -> (16.3837, 2.2184)
  line L145 (16.3837, 2.2184) -> (16.3837, 1.1406)
  line L146 (16.3837, 1.1406) -> (17.5466, 1.1406)
  line L147 (17.5466, 1.1406) -> (17.5466, 0.6179)
  line L148 (17.5466, 0.6179) -> (16.3837, 0.6179)
  line L149 (16.3837, 0.6179) -> (16.3837, -1.169)
  spline S135 degree 2 poles (16.3837, -1.169) (16.3837, -1.4526) (16.404, -1.7646) (16.4729, -1.8983) knots 0 0 0 1 2 2 2
  spline S136 degree 2 poles (16.4729, -1.8983) (16.5296, -2.0158) (16.7848, -2.1333) (17.0036, -2.1333) knots 0 0 0 1 2 2 2
  spline S137 degree 2 poles (17.0036, -2.1333) (17.1576, -2.1333) (17.4453, -2.0401) (17.5101, -2.0118) knots 0 0 0 1 2 2 2
  line L150 (17.5101, -2.0118) -> (17.5466, -2.0118)
  line L151 (17.5466, -2.0118) -> (17.5466, -2.579)
  spline S138 degree 2 poles (17.5466, -2.579) (17.3683, -2.6276) (17.0036, -2.6844) (16.8456, -2.6844) knots 0 0 0 1 2 2 2
  spline S139 degree 2 poles (19.0255, -2.7006) (18.6487, -2.7006) (17.9964, -2.498) (17.7816, -2.3845) knots 0 0 0 1 2 2 2
  line L152 (17.7816, -2.3845) -> (17.7816, -1.6754)
  line L153 (17.7816, -1.6754) -> (17.814, -1.6754)
  spline S140 degree 2 poles (17.814, -1.6754) (17.8951, -1.7403) (18.1139, -1.8942) (18.2962, -1.9793) knots 0 0 0 1 2 2 2
  spline S141 degree 2 poles (18.2962, -1.9793) (18.4542, -2.0563) (18.8432, -2.1698) (19.0498, -2.1698) knots 0 0 0 1 2 2 2
  spline S142 degree 2 poles (19.0498, -2.1698) (19.1998, -2.1698) (19.5442, -2.1009) (19.6252, -2.0442) knots 0 0 0 1 2 2 2
  spline S143 degree 2 poles (19.6252, -2.0442) (19.7427, -1.9672) (19.8481, -1.7929) (19.8481, -1.6147) knots 0 0 0 1 2 2 2
  spline S144 degree 2 poles (19.8481, -1.6147) (19.8481, -1.3918) (19.6049, -1.1609) (19.293, -1.0839) knots 0 0 0 1 2 2 2
  spline S145 degree 2 poles (19.293, -1.0839) (19.1714, -1.0555) (18.7824, -0.9745) (18.6163, -0.9299) knots 0 0 0 1 2 2 2
  spline S146 degree 2 poles (18.6163, -0.9299) (18.1868, -0.8043) (17.7978, -0.2857) (17.7978, 0.0831) knots 0 0 0 1 2 2 2
  spline S147 degree 2 poles (17.7978, 0.0831) (17.7978, 0.5936) (18.5636, 1.2297) (19.1957, 1.2297) knots 0 0 0 1 2 2 2
  spline S148 degree 2 poles (19.1957, 1.2297) (19.5077, 1.2297) (20.1398, 1.0758) (20.3545, 0.9583) knots 0 0 0 1 2 2 2
  line L154 (20.3545, 0.9583) -> (20.3545, 0.2816)
  line L155 (20.3545, 0.2816) -> (20.3221, 0.2816)
  spline S149 degree 2 poles (20.3221, 0.2816) (20.079, 0.4761) (19.4874, 0.6989) (19.1836, 0.6989) knots 0 0 0 1 2 2 2
  spline S150 degree 2 poles (19.1836, 0.6989) (18.8716, 0.6989) (18.4421, 0.4356) (18.4421, 0.1722) knots 0 0 0 1 2 2 2
  spline S151 degree 2 poles (18.4421, 0.1722) (18.4421, -0.0669) (18.6973, -0.2978) (18.981, -0.3707) knots 0 0 0 1 2 2 2
  spline S152 degree 2 poles (18.981, -0.3707) (19.1187, -0.4072) (19.4672, -0.4801) (19.6576, -0.5247) knots 0 0 0 1 2 2 2
  spline S153 degree 2 poles (19.6576, -0.5247) (20.0709, -0.6301) (20.4923, -1.1122) (20.4923, -1.5296) knots 0 0 0 1 2 2 2
  spline S154 degree 2 poles (20.4923, -1.5296) (20.4923, -1.7727) (20.3019, -2.2022) (20.1155, -2.3602) knots 0 0 0 1 2 2 2
  spline S155 degree 2 poles (20.1155, -2.3602) (19.9169, -2.5263) (19.4105, -2.7006) (19.0255, -2.7006) knots 0 0 0 1 2 2 2
  line L156 (-9.9311, -10.8438) -> (-12.3703, -10.8438)
  line L157 (-12.3703, -10.8438) -> (-12.3703, -10.3333)
  line L158 (-12.3703, -10.3333) -> (-11.4627, -10.3333)
  line L159 (-11.4627, -10.3333) -> (-11.4627, -6.9824)
  line L160 (-11.4627, -6.9824) -> (-12.3703, -6.9824)
  line L161 (-12.3703, -6.9824) -> (-12.3703, -6.5245)
  spline S156 degree 2 poles (-12.3703, -6.5245) (-11.8558, -6.5245) (-11.3695, -6.2328) (-11.3371, -5.8276) knots 0 0 0 1 2 2 2
  line L162 (-11.3371, -5.8276) -> (-10.8185, -5.8276)
  line L163 (-10.8185, -5.8276) -> (-10.8185, -10.3333)
  line L164 (-10.8185, -10.3333) -> (-9.9311, -10.3333)
  line L165 (-9.9311, -10.3333) -> (-9.9311, -10.8438)
  line L166 (-4.6637, -10.8438) -> (-4.6637, -8.672)
  spline S157 degree 2 poles (-4.6637, -8.672) (-4.6637, -8.4127) (-4.7042, -7.971) (-4.769, -7.8495) knots 0 0 0 1 2 2 2
  spline S158 degree 2 poles (-4.769, -7.8495) (-4.8339, -7.7158) (-5.081, -7.5861) (-5.2958, -7.5861) knots 0 0 0 1 2 2 2
  spline S159 degree 2 poles (-5.2958, -7.5861) (-5.4903, -7.5861) (-5.936, -7.8252) (-6.171, -8.0521) knots 0 0 0 1 2 2 2
  spline S160 degree 2 poles (-6.171, -8.0521) (-6.1669, -8.1088) (-6.1588, -8.2668) (-6.1588, -8.3722) knots 0 0 0 1 2 2 2
  line L167 (-6.1588, -8.3722) -> (-6.1588, -10.8438)
  line L168 (-6.1588, -10.8438) -> (-6.7909, -10.8438)
  line L169 (-6.7909, -10.8438) -> (-6.7909, -8.672)
  spline S161 degree 2 poles (-6.7909, -8.672) (-6.7909, -8.4127) (-6.8314, -7.971) (-6.8963, -7.8495) knots 0 0 0 1 2 2 2
  spline S162 degree 2 poles (-6.8963, -7.8495) (-6.9611, -7.7158) (-7.2083, -7.5861) (-7.423, -7.5861) knots 0 0 0 1 2 2 2
  spline S163 degree 2 poles (-7.423, -7.5861) (-7.6256, -7.5861) (-8.0754, -7.8414) (-8.2861, -8.0399) knots 0 0 0 1 2 2 2
  line L170 (-8.2861, -8.0399) -> (-8.2861, -10.8438)
  line L171 (-8.2861, -10.8438) -> (-8.9182, -10.8438)
  line L172 (-8.9182, -10.8438) -> (-8.9182, -7.0918)
  line L173 (-8.9182, -7.0918) -> (-8.2861, -7.0918)
  line L174 (-8.2861, -7.0918) -> (-8.2861, -7.5051)
  spline S164 degree 2 poles (-8.2861, -7.5051) (-8.0389, -7.2579) (-7.5527, -6.9864) (-7.2609, -6.9864) knots 0 0 0 1 2 2 2
  spline S165 degree 2 poles (-7.2609, -6.9864) (-6.9287, -6.9864) (-6.4141, -7.2903) (-6.2804, -7.6347) knots 0 0 0 1 2 2 2
  spline S166 degree 2 poles (-6.2804, -7.6347) (-5.9927, -7.3146) (-5.4498, -6.9864) (-5.1337, -6.9864) knots 0 0 0 1 2 2 2
  spline S167 degree 2 poles (-5.1337, -6.9864) (-4.8906, -6.9864) (-4.4935, -7.1363) (-4.3476, -7.3065) knots 0 0 0 1 2 2 2
  spline S168 degree 2 poles (-4.3476, -7.3065) (-4.1977, -7.4767) (-4.0316, -7.9872) (-4.0316, -8.3722) knots 0 0 0 1 2 2 2
  line L175 (-4.0316, -8.3722) -> (-4.0316, -10.8438)
  line L176 (-4.0316, -10.8438) -> (-4.6637, -10.8438)
  line L177 (-2.5, -10.8438) -> (-3.1321, -10.8438)
  line L178 (-3.1321, -10.8438) -> (-3.1321, -5.6209)
  line L179 (-3.1321, -5.6209) -> (-2.5, -5.6209)
  line L180 (-2.5, -5.6209) -> (-2.5, -10.8438)
  line L181 (3.5211, -7.0918) -> (2.107, -10.8438)
  line L182 (2.107, -10.8438) -> (1.5397, -10.8438)
  line L183 (1.5397, -10.8438) -> (0.1378, -7.0918)
  line L184 (0.1378, -7.0918) -> (0.8225, -7.0918)
  line L185 (0.8225, -7.0918) -> (1.8477, -9.9807)
  line L186 (1.8477, -9.9807) -> (2.8647, -7.0918)
  line L187 (2.8647, -7.0918) -> (3.5211, -7.0918)
  line L188 (6.9895, -10.8438) -> (3.906, -10.8438)
  line L189 (3.906, -10.8438) -> (3.906, -10.1347)
  spline S169 degree 2 poles (3.906, -10.1347) (4.2382, -9.8227) (4.8298, -9.2433) (5.1135, -8.9313) knots 0 0 0 1 2 2 2
  spline S170 degree 2 poles (5.1135, -8.9313) (5.6848, -8.3033) (6.1021, -7.5496) (6.1021, -7.1485) knots 0 0 0 1 2 2 2
  spline S171 degree 2 poles (6.1021, -7.1485) (6.1021, -6.9378) (5.9724, -6.6218) (5.8549, -6.5205) knots 0 0 0 1 2 2 2
  spline S172 degree 2 poles (5.8549, -6.5205) (5.7374, -6.4192) (5.4295, -6.3179) (5.2431, -6.3179) knots 0 0 0 1 2 2 2
  spline S173 degree 2 poles (5.2431, -6.3179) (5.0648, -6.3179) (4.7002, -6.407) (4.534, -6.4759) knots 0 0 0 1 2 2 2
  spline S174 degree 2 poles (4.534, -6.4759) (4.3922, -6.5326) (4.1288, -6.6947) (4.0478, -6.7514) knots 0 0 0 1 2 2 2
  line L190 (4.0478, -6.7514) -> (4.0113, -6.7514)
  line L191 (4.0113, -6.7514) -> (4.0113, -6.0383)
  spline S175 degree 2 poles (4.0113, -6.0383) (4.218, -5.937) (4.9595, -5.7384) (5.2917, -5.7384) knots 0 0 0 1 2 2 2
  spline S176 degree 2 poles (5.2917, -5.7384) (5.9927, -5.7384) (6.7828, -6.4799) (6.7828, -7.112) knots 0 0 0 1 2 2 2
  spline S177 degree 2 poles (6.7828, -7.112) (6.7828, -7.4078) (6.6451, -7.9021) (6.5235, -8.1128) knots 0 0 0 1 2 2 2
  spline S178 degree 2 poles (6.5235, -8.1128) (6.4019, -8.3316) (6.0494, -8.7611) (5.8549, -8.9678) knots 0 0 0 1 2 2 2
  spline S179 degree 2 poles (5.8549, -8.9678) (5.5389, -9.3122) (4.765, -10.0496) (4.534, -10.2644) knots 0 0 0 1 2 2 2
  line L192 (4.534, -10.2644) -> (6.9895, -10.2644)
  line L193 (6.9895, -10.2644) -> (6.9895, -10.8438)
  line L194 (8.7318, -10.8438) -> (7.9295, -10.8438)
  line L195 (7.9295, -10.8438) -> (7.9295, -9.8876)
  line L196 (7.9295, -9.8876) -> (8.7318, -9.8876)
  line L197 (8.7318, -9.8876) -> (8.7318, -10.8438)
  line L198 (12.5729, -10.8438) -> (10.1337, -10.8438)
  line L199 (10.1337, -10.8438) -> (10.1337, -10.3333)
  line L200 (10.1337, -10.3333) -> (11.0413, -10.3333)
  line L201 (11.0413, -10.3333) -> (11.0413, -6.9824)
  line L202 (11.0413, -6.9824) -> (10.1337, -6.9824)
  line L203 (10.1337, -6.9824) -> (10.1337, -6.5245)
  spline S180 degree 2 poles (10.1337, -6.5245) (10.6483, -6.5245) (11.1345, -6.2328) (11.1669, -5.8276) knots 0 0 0 1 2 2 2
  line L204 (11.1669, -5.8276) -> (11.6856, -5.8276)
  line L205 (11.6856, -5.8276) -> (11.6856, -10.3333)
  line L206 (11.6856, -10.3333) -> (12.5729, -10.3333)
  line L207 (12.5729, -10.3333) -> (12.5729, -10.8438)
  point P0 (0, 0)
  dimension "d43" = 25
  dimension "d44" = 12.5
  dimension "d45" = 50.8347
  dimension "d46" = 25.4173
  constraints: 2 other
  measures "d43" distance of L2.end L0.start
  measures "d44" distance from line of point (0, 0) L0
  measures "d45" distance of L0.start L0.end
  measures "d46" distance from line of point (0, 0) L3
emboss "Prägen1" sketch "Skizze3" operation cut depth 1 direction (0, 0, -1)
sketch "Skizze4" plane through (0, 0, -7) normal (0, 0, -1) x (-1, 0, 0)
  point P0 (0, 0)
extrude "Extrusion3" add sketch "Skizze1" against normal blind 11 contours A0 E2 L20 L15 L12 L25 | L12 L13 L27 A2 L26 | L31 A3 L23 L14 L15 | L13 L14 L29 A5 E3 L32
chamfer "Fase3" distance 4 angle 45 1 edges at (60.3, 40.85, -5.5)
